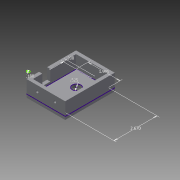
# Autodesk Inventor part: BH_Engineering Club Autonomous Car_Encoder Holder
Saved by Autodesk Inventor 2015 (Build 190159000, 159)
## iProperties
Created: 2015-05-13
Part Number: BH_Engineering Club Autonomous Car_Encoder Holder
Material: Generic
Document SubType Name: Modeling
Designer: 166189
Density: 1 g/cm^3
Appearance: Default
Author: 166189
Autodesk Inventor part; units mm, degrees
ref_plane "YZ Plane" through (0, 0, 0) normal (1, 0, 0) x (0, 1, 0)
ref_plane "XZ Plane" through (0, 0, 0) normal (0, 1, 0) x (-1, 0, 0)
ref_plane "XY Plane" through (0, 0, 0) normal (0, 0, 1) x (1, 0, 0)
sketch "Sketch1" plane through (0, 0, 0) normal (0, 1, 0) x (-1, 0, 0)
  line L0 (0, 0) -> (-50.673, 0)
  line L1 (-50.673, 0) -> (-50.673, -67.818)
  line L2 (-50.673, -67.818) -> (0, -67.818)
  line L3 (0, -67.818) -> (0, 0)
  line L4 (5.08, -72.898) -> (-55.753, -72.898)
  line L5 (-55.753, -72.898) -> (-55.753, 5.08)
  line L6 (-55.753, 5.08) -> (5.08, 5.08)
  line L7 (5.08, 5.08) -> (5.08, -72.898)
  circle A0 centre (-25.019, -43.2562) radius 6.6675
  circle A1 centre (34.7838, -26.9997) radius 2.286
  dimension "d0" = 50.673
  dimension "d1" = 67.818
  dimension "d2" = 5.08
  dimension "d11" = 13.335
  dimension "d14" = 4.572
  constraints: 16 end point, 4 parallel, 2 centre point, 2 perpendicular, 1 horizontal, 4 other
  measures "d0" distance of L2.end L1.end
  measures "d1" distance between parallel lines of L0 L2
  measures "d2" distance between parallel lines of L2 L4
  measures "d11" diameter of A0
  measures "d14" diameter of A1
extrude "Extrusion1" add sketch "Sketch1" along normal blind 20.32 and the other way blind 5.08 contours L4 L5 L6 L7
extrude "Extrusion2" add sketch "Sketch1" against normal blind 5.08 contours L3 L2 L1 L0 | A0
extrude "Extrusion3" cut sketch "Sketch1" against normal blind 127 contours A0
sketch "Sketch2" plane through (-5.08, -5.08, 5.08) normal (-1, 0, 0) x (0, 0, 1)
  line L0 (0, 25.4) -> (-19.685, 25.4)
  line L1 (-77.978, 25.4) -> (0, 25.4) projected
  line L2 (-19.685, 25.4) -> (-19.685, 8.255)
  line L3 (-5.08, 5.08) -> (-72.898, 5.08) projected
  line L4 (-19.685, 8.255) -> (-32.385, 8.255)
  line L5 (-32.385, 8.255) -> (-32.385, 25.4)
  line L6 (-19.685, 25.4) -> (-32.385, 25.4)
  dimension "d15" = 19.685
  dimension "d16" = 17.145
  dimension "d17" = 12.7
  constraints: 10 end point, 3 perpendicular, 2 point on line, 1 collinear
  measures "d15" distance of L0.start L0.end
  measures "d16" distance of L0.end L2.end
  measures "d17" distance of L2.end L4.end
extrude "Extrusion4" cut sketch "Sketch2" against normal blind 25.4
sketch "Sketch5" plane through (-5.08, 20.32, 5.08) normal (0, 0, 1) x (1, 0, 0)
  line L0 (16.51, 0) -> (16.51, -8.89)
  line L1 (0, 0) -> (0, -25.4) projected
  line L2 (60.833, 0) -> (44.323, 0)
  line L3 (0, 0) -> (60.833, 0) projected
  line L4 (44.323, 0) -> (44.323, -8.89)
  circle A0 centre (44.323, -8.89) radius 2.032
  circle A1 centre (16.51, -8.89) radius 2.032
  point P0 (5.08, -20.32)
  point P1 (16.51, -0.0329)
  dimension "d21" = 8.89
  dimension "d22" = 16.51
  dimension "d23" = 16.51
  dimension "d24" = 8.89
  dimension "d25" = 4.064
  dimension "d26" = 4.064
  constraints: 6 end point, 2 centre point, 2 coincident, 2 point on line, 1 perpendicular, 1 vertical
  measures "d21" distance of L0.start L0.end
  measures "d22" distance between parallel lines of L0 L1
  measures "d23" distance of L2.start L2.end
  measures "d24" distance of L2.end L4.end
  measures "d25" diameter of A0
  measures "d26" diameter of A1
extrude "Extrusion5" cut sketch "Sketch5" against normal blind 25.4
body "Solid1"
